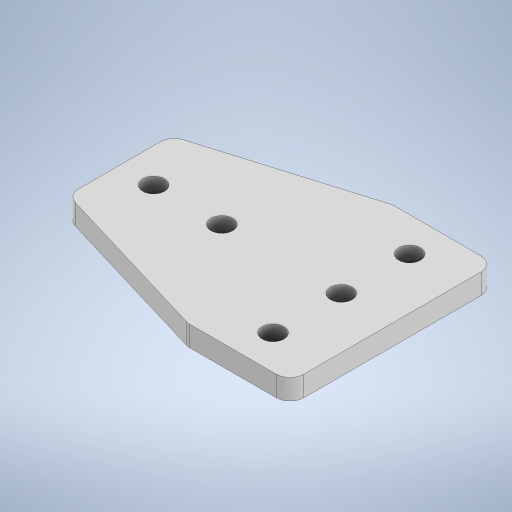
# Autodesk Inventor part: 射出_固定5
Saved by Autodesk Inventor 2023 (Build 270158000, 158)
## iProperties
Created: 2022-04-21
Part Number: 射出_固定5
Material: 一般
Document SubType Name: Modeling
Designer: yuta
Density: 1 g/cm^3
Appearance: 既定
Author: yuta
Autodesk Inventor part; units mm, degrees
ref_plane "YZ Plane" through (0, 0, 0) normal (1, 0, 0) x (0, 1, 0)
ref_plane "XZ Plane" through (0, 0, 0) normal (0, 1, 0) x (-1, 0, 0)
ref_plane "XY Plane" through (0, 0, 0) normal (0, 0, 1) x (1, 0, 0)
sketch "スケッチ1" plane through (0, 0, 0) normal (0, 1, 0) x (-1, 0, 0)
  line L0 (0, 0) -> (15, 0)
  line L1 (40, 0) -> (40, -7.5) construction
  line L2 (40, -30) -> (15, -30) construction
  line L3 (0, -30) -> (0, 0)
  line L4 (40, -7.5) -> (40, -22.5)
  line L5 (40, -7.5) -> (55, -7.5) construction
  line L6 (40, -22.5) -> (15, -30)
  line L7 (40, -7.5) -> (15, 0)
  line L8 (15, 0) -> (40, 0) construction
  line L9 (40, -7.5) -> (40, -22.5)
  line L10 (40, -22.5) -> (40, -30) construction
  line L11 (15, -30) -> (0, -30)
  dimension "d0" = 40
  dimension "d1" = 30
  dimension "d2" = 7.5
  dimension "d3" = 15
  dimension "d4" = 90
  dimension "d5" = 15
  dimension "d6" = 15
  constraints: 24 end point, 7 parallel, 7 perpendicular, 3 collinear, 3 horizontal
  measures "d0" distance of L2.start L3.start
  measures "d1" distance of L1.start L2.start
  measures "d2" distance of L1.start L1.end
  measures "d3" distance of L1.end L4.end
  measures "d4" angle of L4 L5
  measures "d5" distance of L0.start L0.end
  measures "d6" distance of L3.start L2.end
extrude "押し出し1" add sketch "スケッチ1" along normal blind 3
sketch "スケッチ2" plane through (0, 3, 0) normal (0, 1, 0) x (1, 0, 0)
  line L0 (0, 0) -> (0, 30) projected
  line L1 (-15, 0) -> (0, 0) projected
  point P0 (-35, 15)
  point P1 (-35, 15)
  point P2 (-25, 15)
  point P3 (-7.5, 15)
  point P4 (-7.5, 5)
  point P5 (-7.5, 25)
  dimension "d9" = 35
  dimension "d10" = 15
  dimension "d11" = 10
  dimension "d12" = 7.5
  dimension "d13" = 15
  dimension "d14" = 10
  dimension "d15" = 10
  constraints: 1 coincident
  measures "d9" distance from line of L0 point (-35, 15)
  measures "d10" distance from line of L1 point (-35, 15)
  measures "d11" distance of point (-35, 15) point (-25, 15)
  measures "d12" distance from line of L0 point (-7.5, 15)
  measures "d13" distance from line of L1 point (-7.5, 15)
  measures "d14" distance of point (-7.5, 5) point (-7.5, 15)
  measures "d15" distance of point (-7.5, 25) point (-7.5, 15)
hole "穴1" at (-35, 3, -15) at (-25, 3, -15) at (-7.5, 3, -15) at (-7.5, 3, -5) at (-7.5, 3, -25) direction (0, -1, 0) diameter 3.2 end through all
fillet "フィレット1" radius 2 6 edges at (-15, 1.5, 0) (0, 1.5, 0) (0, 1.5, -30) (-40, 1.5, -7.5) (-40, 1.5, -22.5) (-15, 1.5, -30)
